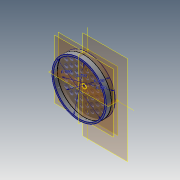
# Autodesk Inventor part: TrayV3
Saved by Autodesk Inventor 2015 (Build 190159000, 159)
## iProperties
Created: 2015-09-29
Part Number: TrayV3
Material: Generic
Document SubType Name: Modeling
Designer: jason
Density: 1 g/cm^3
Appearance: Default
Author: jason
Autodesk Inventor part; units mm, degrees
note: some values were not read from the file. Chosen so that the rebuilt part matches the saved one: second side of "Extrusion5".
sketch "Sketch1" plane through (0, 0, 0) normal (0, 0, 1) x (1, 0, 0)
  circle A0 centre (0, 0) radius 77.216
  circle A1 centre (0, 0) radius 76.2
  dimension "d0" = 154.432
  dimension "d1" = 152.4
  constraints: 2 centre point, 2 coincident
  measures "d0" diameter of A0
  measures "d1" diameter of A1
extrude "Extrusion1" add sketch "Sketch1" along normal blind 2.54 and the other way blind 1.27 contours A1
extrude "Extrusion2" add sketch "Sketch1" along normal blind 25.4
ref_plane "Work Plane1" through (0, 0, 8.4667) normal (0, 0, 1) x (1, 0, 0)
ref_plane "Work Plane2" through (0, 0, 11.0067) normal (0, 0, 1) x (1, 0, 0)
extrude "Extrusion4" add sketch "Sketch1" against normal blind 1.27
sketch "Sketch15" plane through (0, 0, 25.4) normal (0, 0, 1) x (1, 0, 0)
  circle A0 centre (0, 0) radius 77.216
  circle A1 centre (0, 0) radius 73.025
  dimension "d131" = 146.05
  dimension "d140" = 154.432
  constraints: 2 centre point, 2 coincident
  measures "d131" diameter of A1
  measures "d140" diameter of A0
sketch "Sketch8" plane through (0, 0, 8.4667) normal (0, 0, 1) x (1, 0, 0)
  arc A0 (0, -8.4667) -> (0, 8.4667) centre (0, 0) ccw
  arc A1 (0, 8.4667) -> (0, 25.4) centre (0, 16.9333) ccw
  arc A2 (0, -25.4) -> (0, -8.4667) centre (0, -16.9333) ccw
  arc A3 (0, 25.4) -> (0, 42.3333) centre (0, 33.8667) ccw
  arc A4 (0, -42.3333) -> (0, -25.4) centre (0, -33.8667) ccw
  arc A5 (0, 42.3333) -> (0, 59.2667) centre (0, 50.8) ccw
  arc A6 (0, -59.2667) -> (0, -42.3333) centre (0, -50.8) ccw
  arc A7 (0, 59.2667) -> (0, 76.2) centre (0, 67.7333) ccw
  arc A8 (0, -76.2) -> (0, -59.2667) centre (0, -67.7333) ccw
  line L0 (0, 84.1375) -> (0, -84.1375)
  dimension "d31" = 16.9333
  dimension "d32" = 16.9333
  dimension "d33" = 16.9333
  dimension "d34" = 16.9333
  dimension "d35" = 16.9333
  dimension "d36" = 16.9333
  dimension "d38" = 16.9333
  dimension "d39" = 16.9333
  dimension "d40" = 16.9333
  dimension "d41" = 16.9333
  dimension "d42" = 16.9333
  dimension "d43" = 16.9333
  dimension "d44" = 16.9333
  dimension "d45" = 16.9333
  dimension "d46" = 16.9333
  dimension "d47" = 16.9333
  dimension "d48" = 16.9333
  constraints: 18 point on circle, 9 centre point, 1 coincident, 13 other
  measures "d31" diameter of A0
  measures "d32" distance of point (0, 0) A1.centre
  measures "d33" diameter of A1
  measures "d34" diameter of A2
  measures "d35" distance of A2.centre point (0, 0)
  measures "d36" diameter of A3
  measures "d38" distance of A1.centre A3.centre
  measures "d39" distance of A4.centre A2.centre
  measures "d40" diameter of A4
  measures "d41" distance of A3.centre A5.centre
  measures "d42" diameter of A5
  measures "d43" diameter of A6
  measures "d44" distance of A6.centre A4.centre
  measures "d45" diameter of A7
  measures "d46" distance of A5.centre A7.centre
  measures "d47" diameter of A8
  measures "d48" distance of A6.centre A8.centre
revolve "Revolution6" cut sketch "Sketch8" angle 360 about axis through (0, 84.1375, 8.4667) along (0, -1, 0)
sketch "Sketch14" plane through (0, 0, 11.0067) normal (0, 0, 1) x (1, 0, 0)
  circle A0 centre (0, 0) radius 6.0464 projected
  circle A1 centre (0, 0) radius 76.2
  circle A2 centre (0, 0) radius 77.216
  constraints: 2 centre point, 2 coincident
loft "Loft1" add profiles "Sketch14", "Sketch15" contours A0 | A1 | A2 / A0 | A1
loft "Loft2" cut profiles "Sketch14", "Sketch15" contours A0 | A1 / A1
sketch "Sketch9" plane through (0, 0, 8.4667) normal (0, 0, 1) x (1, 0, 0)
  arc A0 (14.6647, 0) -> (14.6647, 16.9333) centre (14.6647, 8.4667) ccw
  line L0 (-30.632, 0) -> (32.868, 0)
  line L1 (0, 84.1375) -> (0, -84.1375)
  arc A1 (14.6647, -16.9333) -> (14.6647, 0) centre (14.6647, -8.4667) ccw
  arc A2 (14.6647, -33.8667) -> (14.6647, -16.9333) centre (14.6647, -25.4) ccw
  arc A3 (14.6647, 16.9333) -> (14.6647, 33.8667) centre (14.6647, 25.4) ccw
  arc A4 (14.6647, 33.8667) -> (14.6647, 50.8) centre (14.6647, 42.3333) ccw
  arc A5 (14.6647, -50.8) -> (14.6647, -33.8667) centre (14.6647, -42.3333) ccw
  arc A6 (14.6647, 50.8) -> (14.6647, 67.7333) centre (14.6647, 59.2667) ccw
  arc A7 (14.6647, -67.7333) -> (14.6647, -50.8) centre (14.6647, -59.2667) ccw
  line L2 (14.6647, 84.1375) -> (14.6647, -84.1375)
  point P0 (0, 0)
  dimension "d53" = 16.9333
  dimension "d54" = 8.4667
  dimension "d55" = 14.6647
  dimension "d56" = 16.9333
  dimension "d57" = 14.6647
  dimension "d58" = 16.9333
  dimension "d59" = 16.9333
  dimension "d60" = 14.6647
  dimension "d61" = 16.9333
  dimension "d62" = 16.9333
  dimension "d63" = 14.6647
  dimension "d64" = 16.9333
  dimension "d65" = 16.9333
  dimension "d68" = 16.9333
  dimension "d69" = 16.9333
  dimension "d70" = 14.6647
  dimension "d71" = 16.9333
  dimension "d72" = 16.9333
  dimension "d73" = 14.6647
  constraints: 16 point on circle, 8 centre point, 4 end point, 12 other
  measures "d53" diameter of A1
  measures "d54" distance from line of L0 A1.centre
  measures "d55" distance from line of L1 A1.centre
  measures "d56" diameter of A2
  measures "d57" distance from line of L1 A2.centre
  measures "d58" distance of A1.centre A2.centre
  measures "d59" diameter of A3
  measures "d60" distance from line of L1 A3.centre
  measures "d61" distance of A0.centre A3.centre
  measures "d62" diameter of A4
  measures "d63" distance from line of L1 A4.centre
  measures "d64" distance of A3.centre A4.centre
  measures "d65" diameter of A5
  measures "d68" diameter of A6
  measures "d69" distance of A4.centre A6.centre
  measures "d70" distance from line of L1 A6.centre
  measures "d71" diameter of A7
  measures "d72" distance of A7.centre A5.centre
  measures "d73" distance from line of L1 A7.centre
revolve "Revolution7" cut sketch "Sketch9" angle 360 about axis through (14.6647, 84.1375, 8.4667) along (0, -1, 0)
sketch "Sketch10" plane through (0, 0, 8.4667) normal (0, 0, 1) x (1, 0, 0)
  arc A0 (29.3294, -8.4667) -> (29.3294, 8.4667) centre (29.3294, 0) ccw
  line L0 (0, 84.1375) -> (0, -84.1375)
  arc A1 (29.3294, 8.4667) -> (29.3294, 25.4) centre (29.3294, 16.9333) ccw
  arc A2 (29.3294, -25.4) -> (29.3294, -8.4667) centre (29.3294, -16.9333) ccw
  arc A3 (29.3294, 25.4) -> (29.3294, 42.3333) centre (29.3294, 33.8667) ccw
  arc A4 (29.3294, -42.3333) -> (29.3294, -25.4) centre (29.3294, -33.8667) ccw
  line L1 (-14.2875, 0) -> (92.075, 0)
  arc A5 (29.3294, 42.3333) -> (29.3294, 59.2667) centre (29.3294, 50.8) ccw
  arc A6 (29.3294, -59.2667) -> (29.3294, -42.3333) centre (29.3294, -50.8) ccw
  line L2 (29.3294, 84.1375) -> (29.3294, -84.1375)
  point P0 (0, 0)
  dimension "d75" = 16.9333
  dimension "d77" = 16.9333
  dimension "d78" = 16.9333
  dimension "d79" = 16.9333
  dimension "d80" = 16.9333
  dimension "d81" = 16.9333
  dimension "d82" = 16.9333
  dimension "d83" = 16.9333
  dimension "d85" = 16.9333
  dimension "d86" = 16.9333
  dimension "d87" = 16.9333
  dimension "d88" = 16.9333
  dimension "d89" = 16.9333
  dimension "d90" = 29.3294
  constraints: 14 point on circle, 7 centre point, 4 end point, 11 other
  measures "d75" diameter of A0
  measures "d77" diameter of A1
  measures "d78" distance of A0.centre A1.centre
  measures "d79" diameter of A2
  measures "d80" distance of A2.centre A0.centre
  measures "d81" diameter of A3
  measures "d82" distance of A1.centre A3.centre
  measures "d83" diameter of A4
  measures "d85" diameter of A5
  measures "d86" distance of A3.centre A5.centre
  measures "d87" diameter of A6
  measures "d88" distance of A6.centre A4.centre
  measures "d89" distance of A4.centre A2.centre
  measures "d90" distance of A0.centre point (0, 0)
revolve "Revolution8" cut sketch "Sketch10" angle 360 about axis through (29.3294, 84.1375, 8.4667) along (0, -1, 0)
sketch "Sketch11" plane through (0, 0, 8.4667) normal (0, 0, 1) x (1, 0, 0)
  arc A0 (43.9941, 0) -> (43.9941, 16.9333) centre (43.9941, 8.4667) ccw
  arc A1 (43.9941, -16.9333) -> (43.9941, 0) centre (43.9941, -8.4667) ccw
  arc A2 (43.9941, 16.9333) -> (43.9941, 33.8667) centre (43.9941, 25.4) ccw
  arc A3 (43.9941, -33.8667) -> (43.9941, -16.9333) centre (43.9941, -25.4) ccw
  arc A4 (43.9941, 33.8667) -> (43.9941, 50.8) centre (43.9941, 42.3333) ccw
  arc A5 (43.9941, -50.8) -> (43.9941, -33.8667) centre (43.9941, -42.3333) ccw
  line L0 (43.9941, 84.1375) -> (43.9941, -84.1375)
  point P0 (0, 0)
  dimension "d92" = 16.9333
  dimension "d93" = 43.9941
  dimension "d94" = 8.4667
  dimension "d95" = 16.9333
  dimension "d96" = 8.4667
  dimension "d97" = 16.9333
  dimension "d98" = 16.9333
  dimension "d99" = 16.9333
  dimension "d100" = 16.9333
  dimension "d101" = 16.9333
  dimension "d102" = 16.9333
  dimension "d103" = 16.9333
  dimension "d104" = 16.9333
  constraints: 12 point on circle, 6 centre point, 10 other
  measures "d92" diameter of A0
  measures "d93" horizontal distance of A0.centre point (0, 0)
  measures "d94" vertical distance of point (0, 0) A0.centre
  measures "d95" diameter of A1
  measures "d96" vertical distance of point (0, 0) A1.centre
  measures "d97" diameter of A2
  measures "d98" distance of A0.centre A2.centre
  measures "d99" diameter of A3
  measures "d100" distance of A3.centre A1.centre
  measures "d101" diameter of A4
  measures "d102" distance of A2.centre A4.centre
  measures "d103" diameter of A5
  measures "d104" distance of A5.centre A3.centre
revolve "Revolution9" cut sketch "Sketch11" angle 360 about axis through (43.9941, 84.1375, 8.4667) along (0, -1, 0)
sketch "Sketch12" plane through (0, 0, 8.4667) normal (0, 0, 1) x (1, 0, 0)
  arc A0 (58.6588, -8.4667) -> (58.6588, 8.4667) centre (58.6588, 0) ccw
  arc A1 (58.6588, 8.4667) -> (58.6588, 25.4) centre (58.6588, 16.9333) ccw
  arc A2 (58.6588, -25.4) -> (58.6588, -8.4667) centre (58.6588, -16.9333) ccw
  arc A3 (58.6588, 25.4) -> (58.6588, 42.3333) centre (58.6588, 33.8667) ccw
  arc A4 (58.6588, -42.3333) -> (58.6588, -25.4) centre (58.6588, -33.8667) ccw
  line L0 (58.6588, 60.325) -> (58.6588, -61.9125)
  point P0 (0, 0)
  dimension "d106" = 16.9333
  dimension "d107" = 58.6588
  dimension "d108" = 16.9333
  dimension "d109" = 16.9333
  dimension "d110" = 16.9333
  dimension "d111" = 16.9333
  dimension "d112" = 16.9333
  dimension "d113" = 16.9333
  dimension "d114" = 16.9333
  dimension "d115" = 16.9333
  constraints: 10 point on circle, 6 point on line, 5 centre point, 2 end point
  measures "d106" diameter of A0
  measures "d107" distance of point (0, 0) A0.centre
  measures "d108" diameter of A1
  measures "d109" diameter of A2
  measures "d110" diameter of A3
  measures "d111" diameter of A4
  measures "d112" distance of A0.centre A1.centre
  measures "d113" distance of A1.centre A3.centre
  measures "d114" distance of A0.centre A2.centre
  measures "d115" distance of A2.centre A4.centre
revolve "Revolution10" cut sketch "Sketch12" angle 360 about axis through (58.6588, 60.325, 8.4667) along (0, -1, 0)
mirror "Mirror1" about plane through (0, 0, 0) normal (1, 0, 0) of "Revolution7", "Revolution8", "Revolution9", "Revolution10"
sketch "Sketch13" plane through (0, 0, 0) normal (0, 0, 1) x (1, 0, 0)
  circle A0 centre (-74.2584, 11.7614) radius 1.016
  circle A1 centre (-74.2584, -11.7614) radius 1.016
  circle A2 centre (-66.9894, -34.1328) radius 1.016
  circle A3 centre (-53.1631, -53.1631) radius 1.016
  circle A4 centre (-34.1328, -66.9894) radius 1.016
  circle A5 centre (-11.7614, -74.2584) radius 1.016
  circle A6 centre (11.7614, -74.2584) radius 1.016
  circle A7 centre (34.1328, -66.9894) radius 1.016
  circle A8 centre (53.1631, -53.1631) radius 1.016
  circle A9 centre (66.9894, -34.1328) radius 1.016
  circle A10 centre (74.2584, -11.7614) radius 1.016
  circle A11 centre (74.2584, 11.7614) radius 1.016
  circle A12 centre (66.9894, 34.1328) radius 1.016
  circle A13 centre (53.1631, 53.1631) radius 1.016
  circle A14 centre (34.1328, 66.9894) radius 1.016
  circle A15 centre (11.7614, 74.2584) radius 1.016
  circle A16 centre (-11.7614, 74.2584) radius 1.016
  circle A17 centre (-34.1328, 66.9894) radius 1.016
  circle A18 centre (-53.1631, 53.1631) radius 1.016
  circle A19 centre (-66.9894, 34.1328) radius 1.016
  circle A20 centre (0, 0) radius 76.2 projected
  circle A21 centre (0, 0) radius 76.2 projected
  line L0 (-74.2584, 11.7614) -> (0, 0)
  circle A22 centre (0, 0) radius 77.216 projected
  line L1 (-84.9518, 0) -> (0, 0)
  dimension "d119" = 2.032
  dimension "d122" = 360
  dimension "d124" = 75.184
  dimension "d129" = 9
  constraints: 20 centre point, 4 end point, 1 horizontal, 41 other
  measures "d119" diameter of A0
  measures "d124" distance of L0.start A20.centre
  measures "d129" angle of L1 L0
extrude "Extrusion5" cut sketch "Sketch13" along normal blind 25.4 contours A0 | A1 | A2 | A3 | A4 | A5 | A6 | A7 | A8 | A9 | A10 | A11 | A12 | A13 | A14 | A15 | A16 | A17 | A18 | A19
equation "\"d32\" = d31"
equation "\"d33\" = d31"
equation "\"d34\" = d31"
equation "\"d35\" = d31"
equation "\"d36\" = d31"
equation "\"d38\" = d31"
equation "\"d39\" = d31"
equation "\"d40\" = d31"
equation "\"d41\" = d31"
equation "\"d42\" = d31"
equation "\"d43\" = d31"
equation "\"d44\" = d31"
equation "\"d45\" = d31"
equation "\"d46\" = d31"
equation "\"d47\" = d31"
equation "\"d48\" = d31"
equation "\"d53\" = d50"
equation "\"d54\" = d51"
equation "\"d55\" = d52"
equation "\"d56\" = d50"
equation "\"d57\" = d55"
equation "\"d58\" = 2 * d54"
equation "\"d59\" = d50"
equation "\"d60\" = d52"
equation "\"d61\" = 2 * d51"
equation "\"d62\" = d50"
equation "\"d63\" = d52"
equation "\"d64\" = d61"
equation "\"d65\" = d53"
equation "\"d68\" = d62"
equation "\"d69\" = d64"
equation "\"d70\" = d60"
equation "\"d71\" = d65"
equation "\"d72\" = d66"
equation "\"d73\" = d67"
equation "\"d77\" = d75"
equation "\"d78\" = d75"
equation "\"d79\" = d75"
equation "\"d80\" = d75"
equation "\"d81\" = d75"
equation "\"d82\" = d75"
equation "\"d83\" = d75"
equation "\"d85\" = d75"
equation "\"d86\" = d75"
equation "\"d87\" = d75"
equation "\"d88\" = d75"
equation "\"d89\" = d75"
equation "\"d95\" = d92"
equation "\"d96\" = 0.5 * d92"
equation "\"d97\" = d92"
equation "\"d98\" = d92"
equation "\"d99\" = d92"
equation "\"d100\" = d92"
equation "\"d101\" = d92"
equation "\"d102\" = d92"
equation "\"d103\" = d92"
equation "\"d104\" = d92"
equation "\"d108\" = d106"
equation "\"d109\" = d106"
equation "\"d110\" = d106"
equation "\"d111\" = d106"
equation "\"d112\" = d106"
equation "\"d113\" = d106"
equation "\"d114\" = d106"
equation "\"d115\" = d106"
equation "\"d51\" = 0.5 * d50"
equation "\"d66\" = d58"
equation "\"d67\" = d57"
equation "\"d50\" = 16.933333"
equation "\"d52\" = 14.664697"
body "Solid1"
